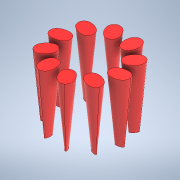
# Autodesk Inventor part: Table Decoration 1
Saved by Autodesk Inventor 2022.4 (Build 264492000, 492)
## iProperties
Created: 2024-05-02
Part Number: Table Decoration 1
Material: Generic
Document SubType Name: Modeling
Designer: t60147996
Density: 1 g/cm^3
Appearance: Light Red
Author: t60147996
Autodesk Inventor part; units mm, degrees
ref_plane "YZ Plane" through (0, 0, 0) normal (1, 0, 0) x (0, 1, 0)
ref_plane "XZ Plane" through (0, 0, 0) normal (0, 1, 0) x (-1, 0, 0)
ref_plane "XY Plane" through (0, 0, 0) normal (0, 0, 1) x (1, 0, 0)
sketch "Sketch1" plane through (0, 0, 0) normal (0, 1, 0) x (-1, 0, 0)
  ellipse E0 centre (12.7, -50.8) end of major axis (16.1229, -56.0973) minor radius 2.2136
  point P0 (0, 0)
  dimension "d0" = 50.8
  dimension "d1" = 12.7
  constraints: 1 centre point
  measures "d0" vertical distance of E0.centre point (0, 0)
  measures "d1" horizontal distance of E0.centre point (0, 0)
extrude "Extrusion1" add sketch "Sketch1" along normal blind 101.6 draft 5
pattern_circular "Circular Pattern1" count 10 over 360 about axis through (0, -10, 0) along (0, 1, 0) of "Extrusion1"
body "Solid1"
